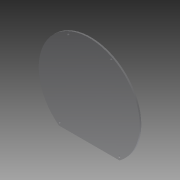
# Autodesk Inventor part: Top Plate
Saved by Autodesk Inventor 2015 (Build 190159000, 159)
## iProperties
Created: 2016-08-02
Part Number: Top Plate
Material: Polycarbonate, Clear
Document SubType Name: Modeling
Designer: James Yelland
Density: 1.2 g/cm^3
Appearance: Polycarbonate - Clear
Author: James Yelland
Autodesk Inventor part; units mm, degrees
ref_plane "YZ Plane" through (0, 0, 0) normal (1, 0, 0) x (0, 1, 0)
ref_plane "XZ Plane" through (0, 0, 0) normal (0, 1, 0) x (-1, 0, 0)
ref_plane "XY Plane" through (0, 0, 0) normal (0, 0, 1) x (1, 0, 0)
sketch "Sketch1" plane through (0, 0, 0) normal (0, 1, 0) x (-1, 0, 0)
  line L0 (0, -80) -> (-60, -80)
  line L1 (0, -80) -> (59.3296, -80)
  arc A0 (60.5404, -79.5918) -> (-60, -80) centre (0, 0) ccw
  arc A1 (59.3296, -80) -> (60.5404, -79.5918) centre (59.3296, -78) ccw
  circle A2 centre (59.0549, -74.4145) radius 1.6
  circle A3 centre (-59.0549, -74.4145) radius 1.6
  circle A4 centre (42.5245, 84.9509) radius 1.6
  circle A5 centre (-42.5245, 84.9509) radius 1.6
  point P0 (60, -80)
  point P1 (0, 0)
  point P2 (0, 0)
  point P3 (0, 0)
  point P4 (0, 0)
  point P5 (0, 0)
  dimension "d2" = 2
  dimension "d5" = 3.2
  dimension "d6" = 3.2
  dimension "d7" = 3.2
  dimension "d8" = 3.2
  constraints: 9 coincident, 6 centre point, 5 point on circle, 4 end point, 2 point on line, 2 tangent
  measures "d2" radius of A1
  measures "d5" diameter of A2
  measures "d6" diameter of A3
  measures "d7" diameter of A4
  measures "d8" diameter of A5
extrude "Extrusion1" add sketch "Sketch1" along normal blind 3
body "Solid1"
